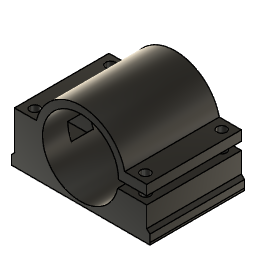
Vexus V.1 (Autodesk Fusion 360 archive; units mm, degrees)
design "BRACKET MOTOR JGA25-370 Rv Version"
Autodesk Fusion 360 part; units mm, degrees
sketch "Sketch1" plane through (0, 0, 0) normal (0, 1, 0) x (1, 0, 0)
  line L0 (-20.9834, -3.1689) -> (-13.9836, -3.2218)
  line L1 (-20.9834, -3.1689) -> (-20.9594, -0.0006)
  line L2 (-21.8983, 10.0959) -> (-20.9045, 9.09)
  line L3 (-20.9045, 9.09) -> (-20.9594, -0.0006)
  line L4 (21, -3.15) -> (21, 0)
  line L5 (21, 9) -> (21, 2.5)
  line L6 (22, 10) -> (21, 9)
  line L7 (22, 12.3548) -> (22, 10)
  line L8 (12.05, 0) -> (21, 0)
  line L9 (11.7878, 2.5) -> (21, 2.5)
  arc A0 (11.7878, 2.5) -> (12.05, 0) centre (0, 0) ccw
  arc A1 (-13.9836, -3.2218) -> (14, -3.15) centre (0, 0) ccw
  line L10 (21, -3.15) -> (14, -3.15)
  line L11 (-21.8983, 10.0959) -> (-21.8983, 13)
  line L12 (-21.8983, 13) -> (22, 13)
  line L13 (22, 13) -> (22, 12.3548)
  dimension "d1" = 24.1
  dimension "d8" = 2.5
  dimension "d61" = 2.3
  dimension "d62" = 135
  dimension "d63" = 135
  dimension "d64" = 1.414
  dimension "d65" = 1.4142
  constraint coincident A0.centre A1.centre
  constraint perpendicular L0 L1
  constraint perpendicular L4 L8
  constraint perpendicular L5 L9
  constraint concentric A0 A1
  constraint perpendicular L4 L10
  constraint vertical L11
  constraint perpendicular L11 L12
  measures "d1" diameter of A0
  measures "d8" distance of L8 L9
  measures "d61" distance of A0 A1
  measures "d62" angle of L5 L6
  measures "d63" angle of L2 L3
  measures "d64" distance of L2.start L2.end
  measures "d65" distance of L5.start L6.start
extrude "Extrude1" add sketch "Sketch1" along normal blind 30
sketch "Sketch3" plane through (-0.0252, 0, 3.3274) normal (-0.007562, 0, 0.999971) x (0, -1, 0)
  circle A0 centre (-27, -17.5) radius 1.5
  circle A1 centre (-3, 17.6) radius 1.5
  circle A2 centre (-27, 17.8) radius 1.5
  circle A3 centre (-3, -17.5) radius 1.5
  dimension "d41" = 3
  dimension "d42" = 3
  dimension "d44" = 3
  measures "d41" diameter of A1
  measures "d42" diameter of A2
  measures "d44" diameter of A3
extrude "Extrude3" cut sketch "Sketch3" against normal blind 19
sketch "Sketch4" plane through (-20.9587, 0, -0.1267) normal (-0.999982, 0, -0.006044) x (0, -1, 0)
  line L0 (0, -8.9635) -> (0, 0.1272)
  line L1 (0, 0.1272) -> (-30, 0.1272)
  line L2 (-30, 0.1272) -> (-30, -8.9635)
  line L3 (-30, -8.9635) -> (0, -8.9635)
  line L4 (-13, 0) -> (-8, 0)
  line L5 (-8, 0) -> (-8, -5)
  line L6 (-19, -7) -> (-24, -7)
  line L7 (-24, -7) -> (-24, -2)
  arc A0 (-22, 0) -> (-24, -2) centre (-22, -2) ccw
  arc A1 (-10, -7) -> (-8, -5) centre (-10, -5) ccw
  line L8 (-15, -2) -> (-15, -7)
  line L9 (-17, 0) -> (-17, -5)
  arc A2 (-19, -7) -> (-17, -5) centre (-19, -5) ccw
  line L10 (-15, -7) -> (-10, -7)
  arc A3 (-13, 0) -> (-15, -2) centre (-13, -2) ccw
  line L11 (-22, 0) -> (-17, 0)
  dimension "d20" = 2
  dimension "d23" = 6
  dimension "d24" = 8
  dimension "d27" = 2
  dimension "d28" = 2
  dimension "d47" = 2
  constraint horizontal L4
  constraint vertical L5
  constraint horizontal L6
  constraint vertical L7
  constraint tangent L4 A0
  constraint tangent L7 A0
  constraint tangent L6 A1
  constraint tangent L5 A1
  constraint equal A0 A1
  constraint coincident L6 A1.start
  constraint tangent L6 A2
  constraint tangent L9 A2
  constraint tangent A1 L10
  constraint coincident L4 A0.start
  constraint tangent L4 A3
  constraint tangent L8 A3
  measures "d20" radius of A0
  measures "d23" distance of L2 L7
  measures "d24" distance of L0 L5
  measures "d27" radius of A2
  measures "d28" radius of A3
  measures "d47" distance of L8 L9
extrude "Extrude5" cut sketch "Sketch4" against normal blind 10 contours L4 L5 A1 L8 L10 A3 | L6 L7 A0 L9 A2 L11
named bodies: "BRACKET MOTOR"
